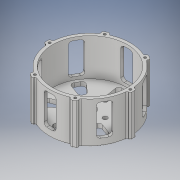
# Autodesk Inventor part: back housing
Saved by Autodesk Inventor 2018 (Build 220112000, 112)
## iProperties
Created: 2019-12-29
Part Number: back housing
Material: Generic
Document SubType Name: Modeling
Designer: mo
Density: 1 g/cm^3
Appearance: Default
Author: mo
## iProperties of the stored document back housing_3DPrint.ipt
Created: 2019-12-29
Part Number: back housing_3DPrint
Material: Generic
Document SubType Name: Modeling
Designer: mo
Density: 1 g/cm^3
Appearance: Default
Author: mo
Autodesk Inventor part; units mm, degrees
ref_plane "YZ Plane" through (0, 0, 0) normal (1, 0, 0) x (0, 1, 0)
ref_plane "XZ Plane" through (0, 0, 0) normal (0, 1, 0) x (-1, 0, 0)
ref_plane "XY Plane" through (0, 0, 0) normal (0, 0, 1) x (1, 0, 0)
sketch "Sketch1" plane through (0, 0, 0) normal (0, 0, 1) x (1, 0, 0)
  circle A0 centre (0, 0) radius 40
  circle A1 centre (0, 0) radius 5.5
  circle A2 centre (0, 0) radius 37
  circle A3 centre (0, 0) radius 8.5
  dimension "d0" = 80
  dimension "d1" = 11
  dimension "d4" = 74
  dimension "d5" = 17
  constraints: 4 centre point, 4 coincident
  measures "d0" diameter of A0
  measures "d1" diameter of A1
  measures "d4" diameter of A2
  measures "d5" diameter of A3
extrude "Extrusion1" add sketch "Sketch1" against normal blind 4 contours A0 | A2 | A3
extrude "Extrusion2" add sketch "Sketch1" along normal blind 37 contours A0
sketch "Sketch2" plane through (0, 0, 0) normal (0, 1, 0) x (-1, 0, 0)
  line L0 (6, 34) -> (-6, 34)
  line L1 (-6, 34) -> (-6, 3)
  line L2 (-6, 3) -> (6, 3)
  line L3 (6, 3) -> (6, 34)
  line L4 (6, 34) -> (-6, 3) construction
  line L5 (-6, 34) -> (6, 3) construction
  line L6 (-56, 0) -> (56, 0) projected
  line L7 (40, 37) -> (-40, 37) projected
  point P0 (0, 0)
  point P1 (0, 18.5)
  dimension "d10" = 3
  dimension "d11" = 3
  dimension "d12" = 12
  constraints: 12 end point, 2 midpoint, 2 parallel, 1 horizontal, 1 perpendicular, 1 vertical alignment
  measures "d10" distance between parallel lines of L6 L2
  measures "d11" distance between parallel lines of L7 L0
  measures "d12" distance between parallel lines of L1 L3
extrude "Extrusion4" cut sketch "Sketch2" along normal through all
sketch "Sketch4" plane through (0, 0, -4) normal (0, 0, -1) x (-1, 0, 0)
  line L0 (43, 3) -> (37, 3)
  line L1 (37, 3) -> (37, -3)
  line L2 (37, -3) -> (43, -3)
  line L3 (43, -3) -> (43, 3)
  line L4 (43, 3) -> (37, -3) construction
  line L5 (37, 3) -> (43, -3) construction
  circle A0 centre (0, 0) radius 37 projected
  point P0 (40, 0)
  point P1 (40, 0)
  dimension "d19" = 6
  dimension "d20" = 6
  constraints: 12 end point, 3 midpoint, 2 horizontal alignment, 2 parallel, 1 horizontal, 1 perpendicular, 1 tangent
  measures "d19" distance of L2.end L0.start
  measures "d20" distance of L1.end L2.end
extrude "Extrusion5" add sketch "Sketch4" against normal up to surface (41 mm away) contours L3 L2 L1 L0
sketch "Sketch5" plane through (0, 0, -4) normal (0, 0, -1) x (-1, 0, 0)
  arc A0 (39.8873, 3) -> (39.8873, -3) centre (0, 0) ccw projected
  point P0 (40, 0)
  constraints: 1 horizontal alignment, 1 point on circle
hole "Hole1" at (-40, 0, -4) direction (0, 0, 1) diameter 2.459 end through all thread size "M3x0.5" class "6H" standard "ISO Metric profile"
fillet "Fillet1" radius 3 4 edges at (6, 38.0289, 3) (6, 38.0289, 34) (-6, 38.0289, 34) (-6, 38.0289, 3)
fillet "Fillet1" radius 1.5 4 edges at (-39.8873, -3, 16.5) (-43, -3, 16.5) (-43, 3, 16.5) (-39.8873, 3, 16.5)
pattern_circular "Circular Pattern1" count 6 over 360 about axis through (0, 0, -10) along (0, 0, 1) of "Fillet1", "Extrusion4", "Extrusion5", "Hole1"
sketch "Sketch8" plane through (0, 0, 0) normal (0, 0, 1) x (1, 0, 0)
  line L0 (0, 0) -> (-5.9951, 34)
  line L1 (-5.9951, 34) -> (5.9951, 34)
  line L2 (5.9951, 34) -> (0, 0)
  line L3 (-3.1739, 18) -> (3.1739, 18)
  dimension "d44" = 20
  dimension "d45" = 16
  dimension "d46" = 18
  constraints: 8 end point, 2 horizontal, 2 point on line, 1 equal length
  measures "d44" angle of L0 L2
  measures "d45" distance between parallel lines of L1 L3
  measures "d46" distance from line of L0.start L3
extrude "Extrusion8" cut sketch "Sketch8" along normal through all both and the other way through all contours L0 L1 L2 L3
fillet "Fillet3" radius 3 4 edges at (5.9951, 34, -2) (-5.9951, 34, -2) (-3.1739, 18, -2) (3.1739, 18, -2)
pattern_circular "Circular Pattern2" count 6 over 360 about axis through (0, 0, -10) along (0, 0, 1) of "Extrusion8", "Fillet3"
fillet "Fillet2" radius 1 48 edges at (23.0569, -33.1692, -4) (23.2869, -34.3341, -4) (23.4979, -35.5783, -4) (21.5, -37.2391, -4) (19.0627, -38.1389, -4) (18.0907, -37.3341, -4) (17.1969, -36.5525, -4) (0, -40, -4) (-17.1969, -36.5525, -4) (-18.0907, -37.3341, -4) (-19.0627, -38.1389, -4) (-21.5, -37.2391, -4) (-23.4979, -35.5783, -4) (-23.2869, -34.3341, -4) (-23.0569, -33.1692, -4) (-34.641, -20, -4) (-40.2538, -3.3833, -4) (-41.3777, -3, -4) (-42.5607, -2.5607, -4) (-43, 0, -4) (-42.5607, 2.5607, -4) (-41.3777, 3, -4) (-40.2538, 3.3833, -4) (-34.641, 20, -4) (0, 40, -4) (34.641, 20, -4) (34.641, -20, -4) (-23.0569, 33.1692, -4) (-23.2869, 34.3341, -4) (-23.4979, 35.5783, -4) (-21.5, 37.2391, -4) (-19.0627, 38.1389, -4) (-18.0907, 37.3341, -4) (-17.1969, 36.5525, -4) (17.1969, 36.5525, -4) (18.0907, 37.3341, -4) (19.0627, 38.1389, -4) (21.5, 37.2391, -4) (23.4979, 35.5783, -4) (23.2869, 34.3341, -4) (23.0569, 33.1692, -4) (40.2538, 3.3833, -4) (41.3777, 3, -4) (42.5607, 2.5607, -4) (43, 0, -4) (42.5607, -2.5607, -4) (41.3777, -3, -4) (40.2538, -3.3833, -4)
sketch "Sketch10" plane through (0, 0, 0) normal (0, 0, 1) x (1, 0, 0)
  point P0 (0, 0)
  point P1 (15, 0)
  dimension "d56" = 15
  constraints: 1 horizontal alignment
  measures "d56" distance of point (0, 0) point (15, 0)
hole "Hole2" at (15, 0, 0) direction (0, 0, -1) diameter 4.5 end through all start extended yes clearance for "Countersunk Flat Head Screw DIN EN ISO 2009" size "M4" standard "DIN"
pattern_circular "Circular Pattern3" count 4 over 360 about axis through (0, 0, -10) along (0, 0, 1) of "Hole2"
body "Solid1"
